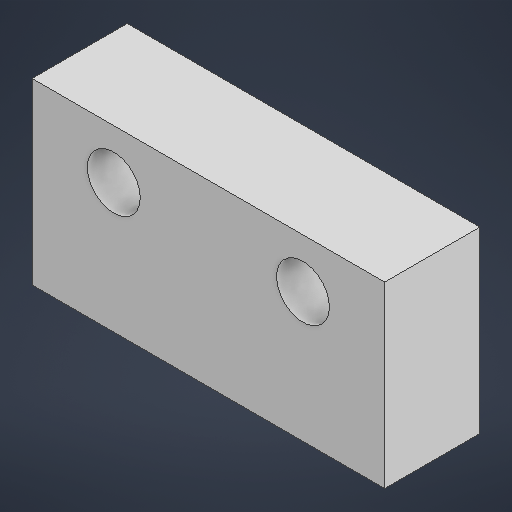
# Autodesk Inventor part: 攻单夹片1
Saved by Autodesk Inventor 2025 (Build 290162000, 162)
## iProperties
Created: 2025-01-08
Part Number: 攻单夹片1
Material: 常规
Document SubType Name: Modeling
Designer: HZD
Density: 1 g/cm^3
Appearance: 默认
Author: HZD
Autodesk Inventor part; units mm, degrees
ref_plane "YZ Plane" through (0, 0, 0) normal (1, 0, 0) x (0, 1, 0)
ref_plane "XZ Plane" through (0, 0, 0) normal (0, 1, 0) x (-1, 0, 0)
ref_plane "XY Plane" through (0, 0, 0) normal (0, 0, 1) x (1, 0, 0)
sketch "草图1" plane through (0, 0, 0) normal (0, 0, 1) x (1, 0, 0)
  line L0 (10, -4.6392) -> (-10, -4.6392)
  line L1 (-10, -4.6392) -> (-10, 5.5)
  line L2 (-10, 5.5) -> (10, 5.5)
  line L3 (10, 5.5) -> (10, -4.6392)
  point P0 (0, 0)
  dimension "d0" = 20
  dimension "d7" = 10.1392
  constraints: 8 end point, 2 parallel, 1 horizontal, 1 perpendicular
  measures "d0" distance of L1.end L2.end
  measures "d7" distance between parallel lines of L2 L0
extrude "拉伸1" add sketch "草图1" along normal blind 5.4
sketch "草图2" plane through (0, 0, 5.4) normal (0, 0, 1) x (1, 0, 0)
  circle A0 centre (-5.3642, 2.7045) radius 1.5 projected
  circle A1 centre (5.3642, 2.7045) radius 1.5 projected
  point P0 (0, 0)
extrude "拉伸2" cut sketch "草图2" against normal blind 21.65
